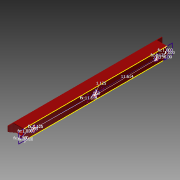
# Autodesk Inventor part: Tube - left
Saved by Autodesk Inventor 2013 (Build 170138000, 138)
## iProperties
Created: 2013-06-28
Part Number: Tube - left
Material: Generic
Document SubType Name: Modeling
Designer: mvarma
Density: 1 g/cm^3
Author: mvarma
Autodesk Inventor part; units mm, degrees
ref_plane "YZ Plane" through (0, 0, 0) normal (1, 0, 0) x (0, 1, 0)
ref_plane "XZ Plane" through (0, 0, 0) normal (0, 1, 0) x (-1, 0, 0)
ref_plane "XY Plane" through (0, 0, 0) normal (0, 0, 1) x (1, 0, 0)
sketch "Sketch1" plane through (0, 0, 0) normal (0, 0, 1) x (1, 0, 0)
  line L0 (0, 0) -> (50.8, 0)
  line L1 (50.8, 0) -> (50.8, 50.8)
  line L2 (50.8, 50.8) -> (0, 50.8)
  line L3 (0, 50.8) -> (0, 0)
  line L4 (3.175, 3.175) -> (47.625, 3.175)
  line L5 (47.625, 3.175) -> (47.625, 47.625)
  line L6 (47.625, 47.625) -> (3.175, 47.625)
  line L7 (3.175, 47.625) -> (3.175, 3.175)
  dimension "d0" = 50.8
  dimension "d1" = 50.8
  dimension "d2" = 44.45
  dimension "d3" = 44.45
  dimension "d4" = 3.175
  dimension "d5" = 3.175
  constraints: 16 end point, 4 parallel, 2 horizontal, 2 perpendicular, 1 coincident
  measures "d0" distance of L2.end L1.end
  measures "d1" distance of L1.end L0.end
  measures "d2" distance of L6.end L5.end
  measures "d3" distance of L5.end L4.end
  measures "d4" distance from line of L0 L4.start
  measures "d5" distance between parallel lines of L3 L7
extrude "Extrusion1" add sketch "Sketch1" along normal blind 736.6
sketch "Sketch2" plane through (50.8, 0, 0) normal (1, 0, 0) x (0, 0, -1)
  line L0 (-736.6, 50.8) -> (-711.2, 50.8)
  line L1 (-711.2, 50.8) -> (-711.2, 25.4)
  line L2 (-711.2, 25.4) -> (-736.6, 25.4)
  line L3 (-736.6, 25.4) -> (-736.6, 50.8)
  line L4 (0, 50.8) -> (-25.4, 50.8)
  line L5 (-25.4, 50.8) -> (-25.4, 25.4)
  line L6 (-25.4, 25.4) -> (0, 25.4)
  line L7 (0, 25.4) -> (0, 50.8)
  line L8 (0, 0) -> (-736.6, 0) projected
  line L9 (-736.6, 25.4) -> (-692.6059, 0)
  line L10 (0, 25.4) -> (-43.9941, 0)
  line L11 (0, 0) -> (0, 50.8) projected
  line L12 (-736.6, 0) -> (-736.6, 50.8) projected
  line L13 (-43.9941, 0) -> (0, 0)
  line L14 (0, 25.4) -> (0, 0)
  line L15 (-736.6, 25.4) -> (-736.6, 0)
  line L16 (-692.6059, 0) -> (-736.6, 0)
  line L17 (0, 50.8) -> (-736.6, 50.8) projected
  line L18 (-736.6, 25.4) -> (0, 25.4) construction
  line L19 (-368.3, 50.8) -> (-368.3, 0) construction
  circle A0 centre (-368.3, 23.8125) radius 14.2875
  circle A1 centre (-73.3171, 26.9875) radius 14.2875
  circle A2 centre (-663.2829, 26.9875) radius 14.2875
  point P0 (-402.9207, 40.0955)
  point P1 (-399.8027, 21.0564)
  point P2 (-338.5841, 34.6282)
  point P3 (-330.0412, 23.8125)
  point P4 (-404.8552, 8.9725)
  point P5 (-428.3922, 43.2675)
  dimension "d8" = 25.4
  dimension "d9" = 25.4
  dimension "d10" = 25.4
  dimension "d11" = 25.4
  dimension "d14" = 30
  dimension "d15" = 30
  dimension "d18" = 28.575
  dimension "d19" = 1.5875
  dimension "d22" = 295
  dimension "d23" = 28.575
  dimension "d24" = 28.575
  dimension "d25" = 295
  dimension "d26" = 1.5875
  dimension "d27" = 1.5875
  constraints: 32 end point, 5 parallel, 3 centre point, 3 perpendicular, 3 point on line, 2 collinear, 2 horizontal, 2 midpoint, 1 coincident, 6 other
  measures "d8" distance of L1.end L2.end
  measures "d9" distance of L0.end L1.end
  measures "d10" distance of L6.end L5.end
  measures "d11" distance of L5.end L4.end
  measures "d14" angle of L8 L10
  measures "d15" angle of L9 L8
  measures "d18" diameter of A0
  measures "d19" distance from line of L18 A0.centre
  measures "d22" distance of A0.centre A2.centre
  measures "d23" diameter of A2
  measures "d24" diameter of A1
  measures "d25" distance of A1.centre A0.centre
  measures "d26" distance from line of L18 A2.centre
  measures "d27" distance from line of L18 A1.centre
extrude "Extrusion2" cut sketch "Sketch2" against normal up to surface (47.625 mm away) contours L0 L1 L2 L3 | L4 L7 L6 L5
extrude "Extrusion3" cut sketch "Sketch2" against normal through all contours L9 L8 L12 | L10 L11 L8
extrude "Extrusion4" cut sketch "Sketch2" against normal through all contours A0 | A1 | A2
hole "Hole1" at (50.8, 40.0955, 402.9207) at (50.8, 8.9725, 404.8552) at (50.8, 23.8125, 330.0412) at (50.8, 43.2675, 428.3922) direction (-1, 0, 0) diameter 9.1281 depth 3.175 tip angle 118
hole "Hole2" at (50.8, 21.0564, 399.8027) at (50.8, 34.6282, 338.5841) direction (-1, 0, 0) diameter 6.5278 depth 25.4 tip angle 118 clearance for "Socket Head Cap Screw" size "1/4" standard "Ansi Unified Screw Threads"
sketch "Sketch3" plane through (3.175, 47.625, 711.2) normal (1, 0, 0) x (0, 0, -1)
  circle A0 centre (311.3973, -26.5686) radius 3.2639 projected
  circle A1 centre (372.6159, -12.9968) radius 3.2639 projected
  point P0 (711.2, -47.625)
hole "Hole3" at (3.175, 21.0564, 399.8027) at (3.175, 34.6282, 338.5841) direction (-1, 0, 0) diameter 10.3188 end through all
equation "\"d8\" = d9"
equation "\"d9\" = d11"
equation "\"d11\" = d10"
equation "\"d15\" = d14"
equation "\"d22\" = d25"
equation "\"d23\" = d18"
equation "\"d24\" = d18"
body "Solid1"
